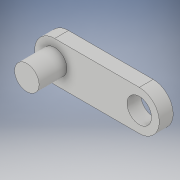
# Autodesk Inventor part: Pedal
Saved by Autodesk Inventor 2019 (Build 230136000, 136)
## iProperties
Created: 2019-11-14
Part Number: Pedal
Material: Generic
Document SubType Name: Modeling
Designer: Domenico
Density: 1 g/cm^3
Appearance: Default
Author: Domenico
Autodesk Inventor part; units mm, degrees
ref_plane "YZ Plane" through (0, 0, 0) normal (1, 0, 0) x (0, 1, 0)
ref_plane "XZ Plane" through (0, 0, 0) normal (0, 1, 0) x (-1, 0, 0)
ref_plane "XY Plane" through (0, 0, 0) normal (0, 0, 1) x (1, 0, 0)
sketch "Sketch1" plane through (0, 0, 0) normal (0, 0, 1) x (1, 0, 0)
  circle A0 centre (0, 0) radius 7.95
  circle A1 centre (-54.9, 0) radius 7.95
  arc A2 (0, -12.95) -> (0, 12.95) centre (0, 0) ccw
  arc A3 (-54.9, 12.95) -> (-54.9, -12.95) centre (-54.9, 0) ccw
  line L0 (-54.2237, 12.95) -> (0, 12.95)
  line L1 (0, -12.95) -> (-54.9, -12.95)
  line L2 (-54.9, 12.95) -> (-54.2237, 12.95)
  dimension "d0" = 15.9
  dimension "d1" = 15.9
  dimension "d2" = 54.9
  dimension "d3" = 5
  dimension "d4" = 5
  dimension "d5" = 54.9
  constraints: 6 end point, 4 centre point, 4 point on circle, 3 coincident, 3 vertical alignment, 1 horizontal, 1 horizontal alignment, 1 parallel
  measures "d0" diameter of A0
  measures "d1" diameter of A1
  measures "d2" distance of point (0, 0) A1.centre
  measures "d3" radial gap between concentric circles of A2 A0
  measures "d4" radial gap between concentric circles of A3 A1
  measures "d5" distance of L1.start L1.end
extrude "Extrusion1" add sketch "Sketch1" along normal blind 9
extrude "Extrusion2" add sketch "Sketch1" along normal blind 27 contours A1
equation "\"d0\" = D_eje"
equation "\"d1\" = D_eje"
equation "\"d4\" = d3"
equation "\"D_eje\" = 15.9"
body "Solid1"
